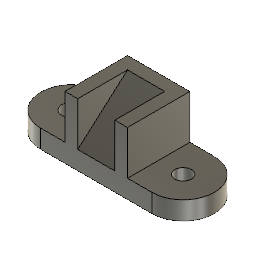
A2 HomeWork 2 (Autodesk Fusion 360 design; units mm, degrees)
Autodesk Fusion 360 part; units mm, degrees
note: some values were not read from the file. Set by a fixed rule: which sketch regions a step uses.
sketch "Sketch1" plane through (0, 0, 0) normal (0, 0, 1) x (1, 0, 0)
  line L0 (0, 0) -> (114, 0)
  line L1 (114, 0) -> (114, 64)
  line L2 (114, 64) -> (0, 64)
  line L3 (0, 64) -> (0, 0)
  dimension "d1" = 114
  dimension "d2" = 64
  constraint horizontal L0
  constraint vertical L1
  constraint horizontal L2
  constraint vertical L3
  constraint coincident L0.start L3.end
  measures "d1" distance of L1 L3
  measures "d2" distance of L0 L2
extrude "Extrude1" add sketch "Sketch1" along normal blind 19
sketch "Sketch2" plane through (0, 0, 19) normal (0, 0, 1) x (-1, 0, 0)
  line L0 (0, -64) -> (0, 0)
  line L1 (0, 0) -> (-114, 0)
  line L2 (-114, 0) -> (-114, -64)
  line L3 (-114, -64) -> (0, -64)
  line L4 (0, 0) -> (-25, 0)
  line L5 (-25, 0) -> (-89, 0)
  line L6 (-89, 0) -> (-89, -64)
  line L7 (-89, -64) -> (-25, -64)
  line L8 (-25, -64) -> (-25, 0)
  dimension "d5" = 25
  dimension "d6" = 64
  constraint coincident L0.end L1.start
  constraint perpendicular L0 L4
  constraint horizontal L5
  constraint vertical L6
  constraint horizontal L7
  constraint vertical L8
  constraint coincident L3 L6.end
  measures "d5" distance of L0.end L4.end
  measures "d6" distance of L6 L8
extrude "Extrude2" add sketch "Sketch2" along normal blind 45 contours L1 L3 L5 L6 L7 L8
sketch "Sketch4" plane through (0, 0, 64) normal (0, 0, 1) x (-1, 0, 0)
  line L0 (-25, -64) -> (-25, 0)
  line L1 (-25, 0) -> (-89, 0)
  line L2 (-89, 0) -> (-89, -64)
  line L3 (-89, -64) -> (-25, -64)
  line L4 (-25, 0) -> (-38, 0)
  line L5 (-38, 0) -> (-38, -51)
  line L6 (-38, -51) -> (-76, -51)
  line L7 (-76, -51) -> (-76, 0)
  line L8 (-38, 0) -> (-76, 0)
  dimension "d12" = 13
  dimension "d13" = 51
  dimension "d14" = 38
  constraint coincident L0.end L1.start
  constraint perpendicular L0 L4
  constraint perpendicular L4 L5
  constraint perpendicular L5 L6
  constraint coincident L1 L7.end
  constraint perpendicular L1 L7
  measures "d12" distance of L0.end L4.end
  measures "d13" distance of L4.end L5.end
  measures "d14" distance of L5.end L6.end
extrude "Extrude3" cut sketch "Sketch4" against normal blind 45 contours L1 L5 L6 L7 L8
sketch "Sketch5" plane through (38, 0, 0) normal (1, 0, 0) x (0, 1, 0)
  line L0 (51, 64) -> (0, 64)
  line L1 (0, 64) -> (0, 19)
  line L2 (0, 19) -> (51, 19)
  line L3 (51, 19) -> (51, 64)
  line L4 (51, 64) -> (0, 19)
  line L5 (51, 19) -> (0, 19)
  line L6 (51, 19) -> (51, 64)
  constraint coincident L0.start L3.end
  constraint coincident L1.end L2.start
  constraint coincident L2.end L3.start
extrude "Extrude4" add sketch "Sketch5" along normal blind 38 contours L2 L3 L4 L5 L6
sketch "Sketch6" plane through (0, 0, 19) normal (0, 0, 1) x (-1, 0, 0)
  line L0 (-89, -64) -> (-89, 0)
  line L1 (-89, 0) -> (-114, 0)
  line L2 (-114, 0) -> (-114, -64)
  line L3 (-114, -64) -> (-89, -64)
  circle A0 centre (-114, -32) radius 32
  line L4 (-114, -64) -> (-114, 0)
  dimension "d31" = 64
  constraint midpoint L2 A0.centre
  constraint coincident L2.end L3.start
  constraint coincident L1.end L2.start
  measures "d31" diameter of A0
extrude "Extrude5" add sketch "Sketch6" against normal blind 19 contours L2 A0 L4
hole "Hole1" at (114, 32, 19) direction (0, 0, -1) diameter 17 depth 22 tip angle 118
sketch "Sketch7" plane through (0, 0, 19) normal (0, 0, 1) x (-1, 0, 0)
  line L0 (-25, 0) -> (-25, -64)
  line L1 (-25, -64) -> (0, -64)
  line L2 (0, -64) -> (0, 0)
  line L3 (0, 0) -> (-25, 0)
  circle A0 centre (0, -32) radius 32
  line L4 (0, -64) -> (0, 0)
  dimension "d25" = 64
  constraint midpoint L2 A0.centre
  constraint coincident L1.end L2.start
  constraint coincident L2.end L3.start
  measures "d25" diameter of A0
extrude "Extrude6" add sketch "Sketch7" against normal blind 19 contours L2 A0 L4
hole "Hole2" at (0, 32, 19) direction (0, 0, -1) diameter 20 depth 22 tip angle 118
